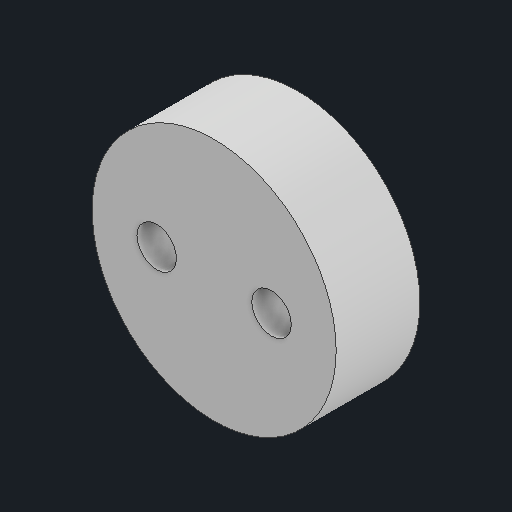
# Autodesk Inventor part: Test_ShaftB
Saved by Autodesk Inventor 2025.1 (Build 291241020, 241B)
## iProperties
Created: 2025-07-24
Part Number: Test_ShaftB
Material: 일반
Document SubType Name: Modeling
Designer: acalo
Density: 1 g/cm^3
Appearance: 기본값
Author: acalo
Autodesk Inventor part; units mm, degrees
ref_plane "YZ Plane" through (0, 0, 0) normal (1, 0, 0) x (0, 1, 0)
ref_plane "XZ Plane" through (0, 0, 0) normal (0, 1, 0) x (-1, 0, 0)
ref_plane "XY Plane" through (0, 0, 0) normal (0, 0, 1) x (1, 0, 0)
sketch "스케치1" plane through (0, 0, 0) normal (0, 0, 1) x (1, 0, 0)
  circle A0 centre (0, 0) radius 10.2
  line L0 (0, 0) -> (4.8, 0)
  line L1 (0, 0) -> (-4.8, 0)
  circle A1 centre (-4.8, 0) radius 1.65
  circle A2 centre (4.8, 0) radius 1.65
  dimension "d0" = 20.4
  dimension "d1" = 4.8
  dimension "d2" = 4.8
  dimension "d3" = 3.3
  dimension "d4" = 3.3
  constraints: 4 end point, 3 centre point, 2 coincident, 2 horizontal
  measures "d0" diameter of A0
  measures "d1" distance of L0.start L0.end
  measures "d2" distance of L0.start L1.end
  measures "d3" diameter of A1
  measures "d4" diameter of A2
extrude "돌출1" add sketch "스케치1" along normal blind 7
